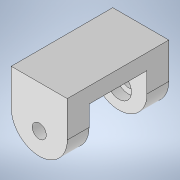
# Autodesk Inventor part: Крепление кулака
Saved by Autodesk Inventor 2020 (Build 240168000, 168)
## iProperties
Created: 2021-06-03
Part Number: Крепление кулака
Material: Типовые
Document SubType Name: Modeling
Designer: Антон
Density: 1 g/cm^3
Appearance: По умолчанию
Author: Антон
Autodesk Inventor part; units mm, degrees
ref_plane "YZ Plane" through (0, 0, 0) normal (1, 0, 0) x (0, 1, 0)
ref_plane "XZ Plane" through (0, 0, 0) normal (0, 1, 0) x (-1, 0, 0)
sketch "Эскиз2" plane through (0, 0, 0) normal (1, 0, 0) x (0, 1, 0)
  line L0 (0, 0) -> (-20.5, 0)
  line L1 (-20.5, 0) -> (-20.5, 32.6)
  line L2 (-20.5, 32.6) -> (0, 32.6)
  line L3 (0, 32.6) -> (0, 0)
  line L4 (-20.5, 0) -> (-20.5, 7)
  line L5 (-20.5, 7) -> (-5, 7)
  line L6 (-5, 7) -> (-5, 25.6)
  line L7 (-5, 25.6) -> (-20.5, 25.6)
  line L8 (-20.5, 25.6) -> (-20.5, 7)
  point P0 (0, 3)
  dimension "d0" = 20.5
  dimension "d1" = 32.6
  dimension "d2" = 7
  dimension "d3" = 15.5
  dimension "d4" = 18.6
  constraints: 18 end point, 4 parallel, 2 horizontal, 2 perpendicular, 2 point on line, 1 coincident
  measures "d0" distance of L1.end L2.end
  measures "d1" distance of L0.end L1.end
  measures "d2" distance of L0.end L4.end
  measures "d3" distance of L7.end L6.end
  measures "d4" distance of L6.end L5.end
extrude "Выдавливание1" add sketch "Эскиз2" along normal blind 18 contours L0 L1 L5 L6 L7 L2 L3
sketch "Эскиз4" plane through (0, -20.5, 32.6) normal (0, 0, 1) x (1, 0, 0)
  line L0 (0, 0) -> (18, 0) projected
  line L1 (9, 0) -> (9, 7)
  circle A0 centre (9, 7) radius 4
  point P0 (0, 20.5)
  dimension "d7" = 7
  dimension "d8" = 8
  constraints: 2 end point, 1 centre point, 1 coincident, 1 midpoint, 1 vertical
  measures "d7" distance of L1.start L1.end
  measures "d8" diameter of A0
extrude "Выдавливание2" cut sketch "Эскиз4" along normal blind 3 from surface at -7
ref_plane "РабПлоскость1" through (18, -5, 16.3) normal (0, 0, -1) x (-1, 0, 0)
mirror "Зеркальное отражение1" about plane through (18, -5, 16.3) normal (0, 0, -1) of "Выдавливание2"
sketch "Эскиз6" plane through (0, -20.5, 32.6) normal (0, 0, 1) x (1, 0, 0)
  circle A0 centre (9, 7) radius 4 projected
  circle A1 centre (9, 7) radius 2.25
  point P0 (0, 20.5)
  dimension "d11" = 4.5
  constraints: 1 centre point, 1 coincident
  measures "d11" diameter of A1
extrude "Выдавливание3" cut sketch "Эскиз6" against normal through all contours A1
fillet "Сопряжение1" radius 9 4 edges at (18, -20.5, 29.1) (0, -20.5, 29.1) (18, -20.5, 3.5) (0, -20.5, 3.5)
equation "\"d2\" = -0.5 * d4 + 0.5 * d1"
